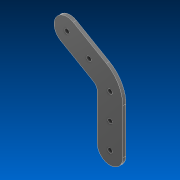
# Autodesk Inventor part: Hood Lower Bracket
Saved by Autodesk Inventor 2022.2 (Build 262287000, 287)
## iProperties
Created: 2022-04-17
Part Number: Hood Lower Bracket
Material: PET Plastic
Document SubType Name: Modeling
Designer: omard
Density: 1.541 g/cm^3
Appearance: Smooth - Black
Author: omard
Autodesk Inventor part; units mm, degrees
ref_plane "YZ Plane" through (0, 0, 0) normal (1, 0, 0) x (0, 1, 0)
ref_plane "XZ Plane" through (0, 0, 0) normal (0, 1, 0) x (-1, 0, 0)
ref_plane "XY Plane" through (0, 0, 0) normal (0, 0, 1) x (1, 0, 0)
sketch "Sketch1" plane through (0, 0, 0) normal (0, 0, 1) x (1, 0, 0)
  line L0 (-12.7, 25.4) -> (12.7, 25.4)
  line L1 (12.7, 25.4) -> (12.7, -25.4)
  line L2 (12.7, -25.4) -> (-12.7, -25.4)
  line L3 (-12.7, -25.4) -> (-12.7, 25.4)
  line L4 (-12.7, 25.4) -> (12.7, -25.4) construction
  line L5 (12.7, 25.4) -> (-12.7, -25.4) construction
  line L6 (-47.6222, 60.6219) -> (-3.6281, 35.2219)
  line L7 (-3.6281, 35.2219) -> (-16.3281, 13.2248)
  line L8 (-16.3281, 13.2248) -> (-60.3222, 38.6248)
  line L9 (-60.3222, 38.6248) -> (-47.6222, 60.6219)
  line L10 (-47.6222, 60.6219) -> (-16.3281, 13.2248) construction
  line L11 (-3.6281, 35.2219) -> (-60.3222, 38.6248) construction
  line L12 (-42.9737, 43.2734) -> (-20.9767, 30.5734) construction
  line L13 (0, -12.7) -> (0, 12.7) construction
  line L14 (-16.3281, 13.2248) -> (-214.3015, 127.5248)
  arc A0 (-12.7, 6.9407) -> (-16.3281, 13.2248) centre (-19.9563, 6.9407) ccw
  arc A1 (12.7, 6.9407) -> (-3.6281, 35.2219) centre (-19.9563, 6.9407) ccw
  line L15 (-12.7, -25.4) -> (12.7, -25.4)
  line L16 (12.7, -25.4) -> (12.7, -50.8)
  line L17 (12.7, -50.8) -> (-12.7, -50.8)
  line L18 (-12.7, -50.8) -> (-12.7, -25.4)
  circle A2 centre (0, -38.1) radius 12.7
  circle A3 centre (-42.9737, 43.2734) radius 12.7
  point P0 (0, 0)
  point P1 (0, 0)
  point P2 (0, 0)
  point P3 (-31.9752, 36.9234)
  point P4 (-31.9752, 36.9234)
  point P5 (-49.3237, 32.2748)
  point P6 (-12.7, -38.1)
  point P7 (12.7, -38.1)
  point P8 (-36.6237, 54.2719)
  dimension "d0" = 25.4
  dimension "d1" = 50.8
  dimension "d2" = 25.4
  dimension "d3" = 12.7
  dimension "d6" = 60
  dimension "d14" = 25.4
  constraints: 38 end point, 8 midpoint, 7 parallel, 6 tangent, 4 centre point, 4 equal length, 4 point on circle, 3 perpendicular, 3 vertical alignment, 2 coincident, 2 horizontal, 2 point on line, 1 collinear, 1 vertical, 3 other
  measures "d0" distance between parallel lines of L3 L1
  measures "d1" distance between parallel lines of L2 L0
  measures "d2" distance of L13.start L13.end
  measures "d3" distance of L13.start point (0, 0)
  measures "d6" angle of L3 L8
  measures "d14" distance of point (0, -38.1) L13.start
extrude "Extrusion1" add sketch "Sketch1" along normal blind 3.175 contours L3 L7 L8 A3 L6 L0 | L0 L7 L3 | L7 A1 L0 | L0 A1 L1 L2 L3 L7 | L3 A0 L7 | A3 | L2 A2 L18 | L16 A2 L2 | A2
hole "Hole1" at (0, -12.7, 0) at (0, 12.7, 0) at (-20.9767, 30.5734, 0) at (-42.9737, 43.2734, 0) at (0, -38.1, 0) direction (0, 0, 1) diameter 4.445 end through all start extended yes
equation "\"d3\" = 0.5 * d2"
equation "\"d14\" = d2"
body "Solid1"
